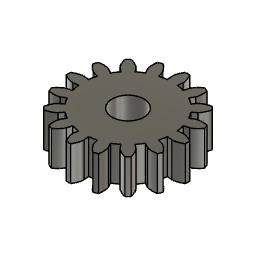
ServoGear v1 (MostComplicated) (Autodesk Fusion 360 design; units mm, degrees)
Autodesk Fusion 360 part; units mm, degrees
note: some values were not read from the file. Set by a fixed rule: which sketch regions a step uses.
sketch "Sketch1" plane through (0, 0, 0) normal (0, 0, 1) x (1, 0, 0) in component "Component"
  spline S0 degree 5 poles (7.171396, -0.814404) (7.171462, -0.814411) (7.171604, -0.814425) (7.171842, -0.814449) (7.172207, -0.814483) (7.172746, -0.814532) (7.173366, -0.814586) (7.174068, -0.814645) (7.174849, -0.814709) (7.175711, -0.814776) (7.176651, -0.814846) (7.177668, -0.814919) (7.178762, -0.814993) (7.179933, -0.815068) (7.181179, -0.815144) (7.1825, -0.81522) (7.183896, -0.815296) (7.185365, -0.815371) (7.186908, -0.815445) (7.188522, -0.815516) (7.190209, -0.815586) (7.191966, -0.815653) (7.193794, -0.815716) (7.195692, -0.815776) (7.197659, -0.815832) (7.199695, -0.815883) (7.201799, -0.815929) (7.20397, -0.815969) (7.206209, -0.816004) (7.208514, -0.816032) (7.210884, -0.816054) (7.21332, -0.816068) (7.215821, -0.816075) (7.218387, -0.816075) (7.221016, -0.816066) (7.223708, -0.816048) (7.226463, -0.816021) (7.22928, -0.815985) (7.232159, -0.81594) (7.235099, -0.815884) (7.2381, -0.815818) (7.241161, -0.815741) (7.244282, -0.815653) (7.247463, -0.815553) (7.250702, -0.815442) (7.254, -0.815319) (7.257356, -0.815183) (7.260769, -0.815035) (7.264239, -0.814874) (7.267766, -0.814699) (7.27135, -0.814511) (7.274989, -0.814309) (7.278683, -0.814093) (7.282432, -0.813863) (7.286236, -0.813617) (7.290094, -0.813357) (7.294006, -0.813081) (7.297971, -0.81279) (7.301989, -0.812483) (7.30606, -0.81216) (7.310182, -0.811821) (7.314357, -0.811465) (7.318582, -0.811092) (7.322859, -0.810702) (7.327187, -0.810294) (7.331564, -0.80987) (7.335991, -0.809427) (7.340468, -0.808966) (7.344994, -0.808487) (7.349569, -0.80799) (7.354192, -0.807474) (7.358863, -0.806939) (7.363582, -0.806384) (7.368349, -0.805811) (7.373162, -0.805217) (7.378022, -0.804604) (7.382928, -0.803971) (7.38788, -0.803318) (7.392878, -0.802644) (7.397921, -0.80195) (7.403009, -0.801235) (7.408142, -0.800498) (7.413319, -0.799741) (7.41854, -0.798962) (7.423805, -0.798162) (7.429113, -0.79734) (7.434465, -0.796495) (7.439859, -0.795629) (7.445295, -0.794741) (7.450774, -0.79383) (7.456294, -0.792896) (7.461856, -0.791939) (7.467459, -0.79096) (7.473103, -0.789957) (7.478788, -0.788931) (7.484513, -0.787882) (7.490278, -0.786808) (7.496083, -0.785711) (7.501927, -0.78459) (7.50781, -0.783445) (7.513733, -0.782276) (7.519693, -0.781082) (7.525693, -0.779864) (7.53173, -0.778621) (7.537805, -0.777353) (7.543917, -0.77606) (7.550067, -0.774741) (7.556253, -0.773398) (7.562476, -0.772029) (7.568736, -0.770635) (7.575032, -0.769214) (7.581363, -0.767768) (7.58773, -0.766296) (7.594133, -0.764798) (7.60057, -0.763274) (7.607042, -0.761723) (7.613549, -0.760146) (7.62009, -0.758542) (7.626666, -0.756911) (7.633274, -0.755254) (7.639917, -0.753569) (7.646593, -0.751858) (7.653301, -0.750119) (7.660043, -0.748353) (7.666817, -0.746559) (7.673623, -0.744738) (7.680462, -0.742889) (7.687332, -0.741013) (7.694233, -0.739108) (7.701166, -0.737176) (7.70813, -0.735215) (7.715125, -0.733226) (7.722151, -0.731209) (7.729207, -0.729164) (7.736292, -0.72709) (7.743408, -0.724987) (7.750554, -0.722856) (7.757729, -0.720696) (7.764933, -0.718507) (7.772166, -0.716289) (7.779428, -0.714041) (7.786718, -0.711765) (7.794037, -0.709459) (7.801383, -0.707124) (7.808758, -0.70476) (7.81616, -0.702366) (7.82359, -0.699942) (7.831046, -0.697489) (7.83853, -0.695006) (7.84604, -0.692493) (7.853577, -0.68995) (7.861141, -0.687376) (7.86873, -0.684773) (7.876345, -0.68214) (7.883986, -0.679476) (7.891653, -0.676782) (7.899344, -0.674057) (7.907061, -0.671302) (7.914802, -0.668516) (7.922568, -0.6657) (7.930359, -0.662853) (7.938173, -0.659975) (7.946012, -0.657066) (7.953875, -0.654126) (7.961761, -0.651156) (7.96967, -0.648154) (7.977603, -0.645121) (7.985558, -0.642056) (7.993537, -0.638961) (8.001538, -0.635834) (8.009561, -0.632675) (8.017607, -0.629485) (8.025674, -0.626264) (8.033764, -0.623011) (8.041874, -0.619726) (8.050007, -0.61641) (8.05816, -0.613062) (8.066335, -0.609681) (8.07453, -0.60627) (8.082746, -0.602826) (8.090983, -0.59935) (8.09924, -0.595842) (8.107516, -0.592301) (8.115813, -0.588729) (8.124129, -0.585124) (8.132465, -0.581488) (8.14082, -0.577818) (8.149195, -0.574117) (8.157588, -0.570383) (8.166, -0.566616) (8.17443, -0.562817) (8.182879, -0.558986) (8.191347, -0.555122) (8.199832, -0.551225) (8.208335, -0.547295) (8.216856, -0.543333) (8.225394, -0.539337) (8.233949, -0.535309) (8.242522, -0.531248) (8.251112, -0.527155) (8.259718, -0.523028) (8.268341, -0.518868) (8.276981, -0.514675) (8.285636, -0.510449) (8.294308, -0.50619) (8.302996, -0.501898) (8.311699, -0.497572) (8.320418, -0.493213) (8.329153, -0.488821) (8.337902, -0.484396) (8.346667, -0.479937) (8.355446, -0.475445) (8.36424, -0.47092) (8.373049, -0.466361) (8.381872, -0.461768) (8.39071, -0.457142) (8.399561, -0.452483) (8.408426, -0.44779) (8.417305, -0.443063) (8.426198, -0.438303) (8.435104, -0.433509) (8.444023, -0.428681) (8.452955, -0.42382) (8.4619, -0.418925) (8.470857, -0.413996) (8.479828, -0.409033) (8.48881, -0.404036) (8.497805, -0.399006) (8.506812, -0.393942) (8.515831, -0.388844) (8.524862, -0.383711) (8.533904, -0.378545) (8.542958, -0.373345) (8.552023, -0.368111) (8.561099, -0.362843) (8.570186, -0.357541) (8.579284, -0.352205) (8.588392, -0.346835) (8.597511, -0.341431) (8.60664, -0.335992) (8.615779, -0.33052) (8.623099, -0.326114) (8.628594, -0.322795) (8.632259, -0.320575) (8.634092, -0.319464) knots 0 0 0 0 0 0 0.00416667 0.00833333 0.0125 0.01666667 0.02083333 0.025 0.02916667 0.03333333 0.0375 0.04166667 0.04583333 0.05 0.05416667 0.05833333 0.0625 0.06666667 0.07083333 0.075 0.07916667 0.08333333 0.0875 0.09166667 0.09583333 0.1 0.10416667 0.10833333 0.1125 0.11666667 0.12083333 0.125 0.12916667 0.13333333 0.1375 0.14166667 0.14583333 0.15 0.15416667 0.15833333 0.1625 0.16666667 0.17083333 0.175 0.17916667 0.18333333 0.1875 0.19166667 0.19583333 0.2 0.20416667 0.20833333 0.2125 0.21666667 0.22083333 0.225 0.22916667 0.23333333 0.2375 0.24166667 0.24583333 0.25 0.25416667 0.25833333 0.2625 0.26666667 0.27083333 0.275 0.27916667 0.28333333 0.2875 0.29166667 0.29583333 0.3 0.30416667 0.30833333 0.3125 0.31666667 0.32083333 0.325 0.32916667 0.33333333 0.3375 0.34166667 0.34583333 0.35 0.35416667 0.35833333 0.3625 0.36666667 0.37083333 0.375 0.37916667 0.38333333 0.3875 0.39166667 0.39583333 0.4 0.40416667 0.40833333 0.4125 0.41666667 0.42083333 0.425 0.42916667 0.43333333 0.4375 0.44166667 0.44583333 0.45 0.45416667 0.45833333 0.4625 0.46666667 0.47083333 0.475 0.47916667 0.48333333 0.4875 0.49166667 0.49583333 0.5 0.50416667 0.50833333 0.5125 0.51666667 0.52083333 0.525 0.52916667 0.53333333 0.5375 0.54166667 0.54583333 0.55 0.55416667 0.55833333 0.5625 0.56666667 0.57083333 0.575 0.57916667 0.58333333 0.5875 0.59166667 0.59583333 0.6 0.60416667 0.60833333 0.6125 0.61666667 0.62083333 0.625 0.62916667 0.63333333 0.6375 0.64166667 0.64583333 0.65 0.65416667 0.65833333 0.6625 0.66666667 0.67083333 0.675 0.67916667 0.68333333 0.6875 0.69166667 0.69583333 0.7 0.70416667 0.70833333 0.7125 0.71666667 0.72083333 0.725 0.72916667 0.73333333 0.7375 0.74166667 0.74583333 0.75 0.75416667 0.75833333 0.7625 0.76666667 0.77083333 0.775 0.77916667 0.78333333 0.7875 0.79166667 0.79583333 0.8 0.80416667 0.80833333 0.8125 0.81666667 0.82083333 0.825 0.82916667 0.83333333 0.8375 0.84166667 0.84583333 0.85 0.85416667 0.85833333 0.8625 0.86666667 0.87083333 0.875 0.87916667 0.88333333 0.8875 0.89166667 0.89583333 0.9 0.90416667 0.90833333 0.9125 0.91666667 0.92083333 0.925 0.92916667 0.93333333 0.9375 0.94166667 0.94583333 0.95 0.95416667 0.95833333 0.9625 0.96666667 0.97083333 0.975 0.97916667 0.98333333 0.9875 0.99166667 0.99583333 1 1 1 1 1 1
  spline S1 degree 5 poles (7.171396, 0.814404) (7.171462, 0.814411) (7.171604, 0.814425) (7.171842, 0.814449) (7.172207, 0.814483) (7.172746, 0.814532) (7.173366, 0.814586) (7.174068, 0.814645) (7.174849, 0.814709) (7.175711, 0.814776) (7.176651, 0.814846) (7.177668, 0.814919) (7.178762, 0.814993) (7.179933, 0.815068) (7.181179, 0.815144) (7.1825, 0.81522) (7.183896, 0.815296) (7.185365, 0.815371) (7.186908, 0.815445) (7.188522, 0.815516) (7.190209, 0.815586) (7.191966, 0.815653) (7.193794, 0.815716) (7.195692, 0.815776) (7.197659, 0.815832) (7.199695, 0.815883) (7.201799, 0.815929) (7.20397, 0.815969) (7.206209, 0.816004) (7.208514, 0.816032) (7.210884, 0.816054) (7.21332, 0.816068) (7.215821, 0.816075) (7.218387, 0.816075) (7.221016, 0.816066) (7.223708, 0.816048) (7.226463, 0.816021) (7.22928, 0.815985) (7.232159, 0.81594) (7.235099, 0.815884) (7.2381, 0.815818) (7.241161, 0.815741) (7.244282, 0.815653) (7.247463, 0.815553) (7.250702, 0.815442) (7.254, 0.815319) (7.257356, 0.815183) (7.260769, 0.815035) (7.264239, 0.814874) (7.267766, 0.814699) (7.27135, 0.814511) (7.274989, 0.814309) (7.278683, 0.814093) (7.282432, 0.813863) (7.286236, 0.813617) (7.290094, 0.813357) (7.294006, 0.813081) (7.297971, 0.81279) (7.301989, 0.812483) (7.30606, 0.81216) (7.310182, 0.811821) (7.314357, 0.811465) (7.318582, 0.811092) (7.322859, 0.810702) (7.327187, 0.810294) (7.331564, 0.80987) (7.335991, 0.809427) (7.340468, 0.808966) (7.344994, 0.808487) (7.349569, 0.80799) (7.354192, 0.807474) (7.358863, 0.806939) (7.363582, 0.806384) (7.368349, 0.805811) (7.373162, 0.805217) (7.378022, 0.804604) (7.382928, 0.803971) (7.38788, 0.803318) (7.392878, 0.802644) (7.397921, 0.80195) (7.403009, 0.801235) (7.408142, 0.800498) (7.413319, 0.799741) (7.41854, 0.798962) (7.423805, 0.798162) (7.429113, 0.79734) (7.434465, 0.796495) (7.439859, 0.795629) (7.445295, 0.794741) (7.450774, 0.79383) (7.456294, 0.792896) (7.461856, 0.791939) (7.467459, 0.79096) (7.473103, 0.789957) (7.478788, 0.788931) (7.484513, 0.787882) (7.490278, 0.786808) (7.496083, 0.785711) (7.501927, 0.78459) (7.50781, 0.783445) (7.513733, 0.782276) (7.519693, 0.781082) (7.525693, 0.779864) (7.53173, 0.778621) (7.537805, 0.777353) (7.543917, 0.77606) (7.550067, 0.774741) (7.556253, 0.773398) (7.562476, 0.772029) (7.568736, 0.770635) (7.575032, 0.769214) (7.581363, 0.767768) (7.58773, 0.766296) (7.594133, 0.764798) (7.60057, 0.763274) (7.607042, 0.761723) (7.613549, 0.760146) (7.62009, 0.758542) (7.626666, 0.756911) (7.633274, 0.755254) (7.639917, 0.753569) (7.646593, 0.751858) (7.653301, 0.750119) (7.660043, 0.748353) (7.666817, 0.746559) (7.673623, 0.744738) (7.680462, 0.742889) (7.687332, 0.741013) (7.694233, 0.739108) (7.701166, 0.737176) (7.70813, 0.735215) (7.715125, 0.733226) (7.722151, 0.731209) (7.729207, 0.729164) (7.736292, 0.72709) (7.743408, 0.724987) (7.750554, 0.722856) (7.757729, 0.720696) (7.764933, 0.718507) (7.772166, 0.716289) (7.779428, 0.714041) (7.786718, 0.711765) (7.794037, 0.709459) (7.801383, 0.707124) (7.808758, 0.70476) (7.81616, 0.702366) (7.82359, 0.699942) (7.831046, 0.697489) (7.83853, 0.695006) (7.84604, 0.692493) (7.853577, 0.68995) (7.861141, 0.687376) (7.86873, 0.684773) (7.876345, 0.68214) (7.883986, 0.679476) (7.891653, 0.676782) (7.899344, 0.674057) (7.907061, 0.671302) (7.914802, 0.668516) (7.922568, 0.6657) (7.930359, 0.662853) (7.938173, 0.659975) (7.946012, 0.657066) (7.953875, 0.654126) (7.961761, 0.651156) (7.96967, 0.648154) (7.977603, 0.645121) (7.985558, 0.642056) (7.993537, 0.638961) (8.001538, 0.635834) (8.009561, 0.632675) (8.017607, 0.629485) (8.025674, 0.626264) (8.033764, 0.623011) (8.041874, 0.619726) (8.050007, 0.61641) (8.05816, 0.613062) (8.066335, 0.609681) (8.07453, 0.60627) (8.082746, 0.602826) (8.090983, 0.59935) (8.09924, 0.595842) (8.107516, 0.592301) (8.115813, 0.588729) (8.124129, 0.585124) (8.132465, 0.581488) (8.14082, 0.577818) (8.149195, 0.574117) (8.157588, 0.570383) (8.166, 0.566616) (8.17443, 0.562817) (8.182879, 0.558986) (8.191347, 0.555122) (8.199832, 0.551225) (8.208335, 0.547295) (8.216856, 0.543333) (8.225394, 0.539337) (8.233949, 0.535309) (8.242522, 0.531248) (8.251112, 0.527155) (8.259718, 0.523028) (8.268341, 0.518868) (8.276981, 0.514675) (8.285636, 0.510449) (8.294308, 0.50619) (8.302996, 0.501898) (8.311699, 0.497572) (8.320418, 0.493213) (8.329153, 0.488821) (8.337902, 0.484396) (8.346667, 0.479937) (8.355446, 0.475445) (8.36424, 0.47092) (8.373049, 0.466361) (8.381872, 0.461768) (8.39071, 0.457142) (8.399561, 0.452483) (8.408426, 0.44779) (8.417305, 0.443063) (8.426198, 0.438303) (8.435104, 0.433509) (8.444023, 0.428681) (8.452955, 0.42382) (8.4619, 0.418925) (8.470857, 0.413996) (8.479828, 0.409033) (8.48881, 0.404036) (8.497805, 0.399006) (8.506812, 0.393942) (8.515831, 0.388844) (8.524862, 0.383711) (8.533904, 0.378545) (8.542958, 0.373345) (8.552023, 0.368111) (8.561099, 0.362843) (8.570186, 0.357541) (8.579284, 0.352205) (8.588392, 0.346835) (8.597511, 0.341431) (8.60664, 0.335992) (8.615779, 0.33052) (8.623099, 0.326114) (8.628594, 0.322795) (8.632259, 0.320575) (8.634092, 0.319464) knots 0 0 0 0 0 0 0.00416667 0.00833333 0.0125 0.01666667 0.02083333 0.025 0.02916667 0.03333333 0.0375 0.04166667 0.04583333 0.05 0.05416667 0.05833333 0.0625 0.06666667 0.07083333 0.075 0.07916667 0.08333333 0.0875 0.09166667 0.09583333 0.1 0.10416667 0.10833333 0.1125 0.11666667 0.12083333 0.125 0.12916667 0.13333333 0.1375 0.14166667 0.14583333 0.15 0.15416667 0.15833333 0.1625 0.16666667 0.17083333 0.175 0.17916667 0.18333333 0.1875 0.19166667 0.19583333 0.2 0.20416667 0.20833333 0.2125 0.21666667 0.22083333 0.225 0.22916667 0.23333333 0.2375 0.24166667 0.24583333 0.25 0.25416667 0.25833333 0.2625 0.26666667 0.27083333 0.275 0.27916667 0.28333333 0.2875 0.29166667 0.29583333 0.3 0.30416667 0.30833333 0.3125 0.31666667 0.32083333 0.325 0.32916667 0.33333333 0.3375 0.34166667 0.34583333 0.35 0.35416667 0.35833333 0.3625 0.36666667 0.37083333 0.375 0.37916667 0.38333333 0.3875 0.39166667 0.39583333 0.4 0.40416667 0.40833333 0.4125 0.41666667 0.42083333 0.425 0.42916667 0.43333333 0.4375 0.44166667 0.44583333 0.45 0.45416667 0.45833333 0.4625 0.46666667 0.47083333 0.475 0.47916667 0.48333333 0.4875 0.49166667 0.49583333 0.5 0.50416667 0.50833333 0.5125 0.51666667 0.52083333 0.525 0.52916667 0.53333333 0.5375 0.54166667 0.54583333 0.55 0.55416667 0.55833333 0.5625 0.56666667 0.57083333 0.575 0.57916667 0.58333333 0.5875 0.59166667 0.59583333 0.6 0.60416667 0.60833333 0.6125 0.61666667 0.62083333 0.625 0.62916667 0.63333333 0.6375 0.64166667 0.64583333 0.65 0.65416667 0.65833333 0.6625 0.66666667 0.67083333 0.675 0.67916667 0.68333333 0.6875 0.69166667 0.69583333 0.7 0.70416667 0.70833333 0.7125 0.71666667 0.72083333 0.725 0.72916667 0.73333333 0.7375 0.74166667 0.74583333 0.75 0.75416667 0.75833333 0.7625 0.76666667 0.77083333 0.775 0.77916667 0.78333333 0.7875 0.79166667 0.79583333 0.8 0.80416667 0.80833333 0.8125 0.81666667 0.82083333 0.825 0.82916667 0.83333333 0.8375 0.84166667 0.84583333 0.85 0.85416667 0.85833333 0.8625 0.86666667 0.87083333 0.875 0.87916667 0.88333333 0.8875 0.89166667 0.89583333 0.9 0.90416667 0.90833333 0.9125 0.91666667 0.92083333 0.925 0.92916667 0.93333333 0.9375 0.94166667 0.94583333 0.95 0.95416667 0.95833333 0.9625 0.96666667 0.97083333 0.975 0.97916667 0.98333333 0.9875 0.99166667 0.99583333 1 1 1 1 1 1
  spline S2 degree 5 poles (7.170748, -0.814336) (7.170774, -0.814339) (7.170826, -0.814344) (7.170903, -0.814352) (7.171007, -0.814363) (7.171137, -0.814377) (7.17124, -0.814387) (7.171318, -0.814396) (7.17137, -0.814401) (7.171396, -0.814404) knots 0 0 0 0 0 0 0.2 0.4 0.6 0.8 1 1 1 1 1 1
  spline S3 degree 5 poles (7.170748, 0.814336) (7.170774, 0.814339) (7.170826, 0.814344) (7.170903, 0.814352) (7.171007, 0.814363) (7.171137, 0.814377) (7.17124, 0.814387) (7.171318, 0.814396) (7.17137, 0.814401) (7.171396, 0.814404) knots 0 0 0 0 0 0 0.2 0.4 0.6 0.8 1 1 1 1 1 1
  line L0 (0, 0) -> (7.170748, -0.814336)
  line L1 (0, 0) -> (7.170748, 0.814336)
  arc A0 (8.634092, -0.319464) -> (8.634092, 0.319464) centre (0, 0) ccw
  point P0 (7.173341, -0.814584)
  point P1 (7.176587, -0.814841)
  point P2 (7.181135, -0.81514)
  point P3 (7.186988, -0.815447)
  point P4 (7.194145, -0.815726)
  point P5 (7.202608, -0.815943)
  point P6 (7.212374, -0.816062)
  point P7 (7.223444, -0.816048)
  point P8 (7.235815, -0.815867)
  point P9 (7.249485, -0.815483)
  point P10 (7.264449, -0.814861)
  point P11 (7.280704, -0.813967)
  point P12 (7.298244, -0.812767)
  point P13 (7.317065, -0.811224)
  point P14 (7.33716, -0.809305)
  point P15 (7.358522, -0.806975)
  point P16 (7.381144, -0.804199)
  point P17 (7.405017, -0.800945)
  point P18 (7.430131, -0.797176)
  point P19 (7.456478, -0.792861)
  point P20 (7.484047, -0.787964)
  point P21 (7.512827, -0.782452)
  point P22 (7.542806, -0.776292)
  point P23 (7.573972, -0.76945)
  point P24 (7.606311, -0.761895)
  point P25 (7.639809, -0.753592)
  point P26 (7.674453, -0.74451)
  point P27 (7.710228, -0.734616)
  point P28 (7.747116, -0.723879)
  point P29 (7.785102, -0.712266)
  point P30 (7.824169, -0.699747)
  point P31 (7.8643, -0.68629)
  point P32 (7.905475, -0.671865)
  point P33 (7.947675, -0.656441)
  point P34 (7.990882, -0.639987)
  point P35 (8.035075, -0.622476)
  point P36 (8.080233, -0.603876)
  point P37 (8.126334, -0.584159)
  point P38 (8.173356, -0.563297)
  point P39 (8.221278, -0.54126)
  point P40 (8.270075, -0.518022)
  point P41 (8.319723, -0.493555)
  point P42 (8.370199, -0.467832)
  point P43 (8.421477, -0.440827)
  point P44 (8.473532, -0.412512)
  point P45 (8.526337, -0.382864)
  point P46 (8.579866, -0.351856)
  point P47 (7.173341, 0.814584)
  point P48 (7.176587, 0.814841)
  point P49 (7.181135, 0.81514)
  point P50 (7.186988, 0.815447)
  point P51 (7.194145, 0.815726)
  point P52 (7.202608, 0.815943)
  point P53 (7.212374, 0.816062)
  point P54 (7.223444, 0.816048)
  point P55 (7.235815, 0.815867)
  point P56 (7.249485, 0.815483)
  point P57 (7.264449, 0.814861)
  point P58 (7.280704, 0.813967)
  point P59 (7.298244, 0.812767)
  point P60 (7.317065, 0.811224)
  point P61 (7.33716, 0.809305)
  point P62 (7.358522, 0.806975)
  point P63 (7.381144, 0.804199)
  point P64 (7.405017, 0.800945)
  point P65 (7.430131, 0.797176)
  point P66 (7.456478, 0.792861)
  point P67 (7.484047, 0.787964)
  point P68 (7.512827, 0.782452)
  point P69 (7.542806, 0.776292)
  point P70 (7.573972, 0.76945)
  point P71 (7.606311, 0.761895)
  point P72 (7.639809, 0.753592)
  point P73 (7.674453, 0.74451)
  point P74 (7.710228, 0.734616)
  point P75 (7.785102, 0.712266)
  point P76 (7.824169, 0.699747)
  point P77 (7.8643, 0.68629)
  point P78 (7.905475, 0.671865)
  point P79 (7.947675, 0.656441)
  point P80 (7.990882, 0.639987)
  point P81 (8.035075, 0.622476)
  point P82 (8.080233, 0.603876)
  point P83 (8.126334, 0.584159)
  point P84 (8.173356, 0.563297)
  point P85 (8.221278, 0.54126)
  point P86 (8.270075, 0.518022)
  point P87 (8.319723, 0.493555)
  point P88 (8.370199, 0.467832)
  point P89 (8.421477, 0.440827)
  point P90 (8.473532, 0.412512)
  point P91 (8.526337, 0.382864)
  point P92 (8.579866, 0.351856)
sketch "Sketch2" plane through (0, 0, 0) normal (0, 0, 1) x (1, 0, 0) in component "Component"
  circle A0 centre (0, 0) radius 6.48
extrude "Extrude1" add sketch "Sketch2" along normal blind 5 makes body 1 in component "Component"
extrude "Extrude2" add sketch "Sketch1" along normal blind 5 separate body makes body 2 in component "Component"
pattern_circular "C-Pattern1" count 16 over 360 about axis through (0, 0, 1.75) along (0, 0, 1) of "Extrude2" makes body 3 makes body 4 makes body 5 makes body 6 makes body 7 makes body 8 makes body 9 makes body 10 makes body 11 makes body 12 makes body 13 makes body 14 makes body 15 makes body 16 makes body 17 in component "Component"
combine "Combine1" operation add target body 1 tool bodies 2 3 4 5 6 7 8 9 10 11 12 13 14 15 16 17 in component "Component"
sketch "Sketch3" plane through (0, 0, 0) normal (0, 0, 1) x (1, 0, 0) in component "Component"
  line L0 (0, 0) -> (50.843263, 0) construction
  line L1 (50.843263, 0) -> (50.843263, 3) construction
  line L2 (50.843263, 3) -> (0, 3) construction
  line L3 (0, 3) -> (0, 0) construction
  constraint perpendicular L0 L1
  constraint parallel L0 L2
  constraint parallel L1 L3
cylinder "CylinderPrimitive1" cut diameter 4.6 height 4 placed x (1, 0, 0) y (0, 1, 0) z (0, 0, 1) at (0, 0, 0) bodies 1 in component "Component"
component "Component" placed x (1, 0, 0) y (0, 1, 0) z (0, 0, 1) at (0, 0, 0)
